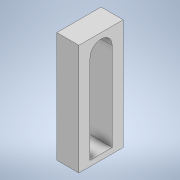
# Autodesk Inventor part: 뚫린 직육면체
Saved by Autodesk Inventor 2022 (Build 260153000, 153)
## iProperties
Created: 2022-10-28
Part Number: 뚫린 직육면체
Material: 일반
Document SubType Name: Modeling
Designer: gogin
Density: 1 g/cm^3
Appearance: 기본값
Author: gogin
Autodesk Inventor part; units mm, degrees
ref_plane "YZ Plane" through (0, 0, 0) normal (1, 0, 0) x (0, 1, 0)
ref_plane "XZ Plane" through (0, 0, 0) normal (0, 1, 0) x (-1, 0, 0)
ref_plane "XY Plane" through (0, 0, 0) normal (0, 0, 1) x (1, 0, 0)
sketch "스케치1" plane through (0, 0, 0) normal (1, 0, 0) x (0, 1, 0)
  line L0 (4.5, 0) -> (-0.5, 0)
  line L1 (-0.5, 0) -> (-0.5, -2)
  line L2 (-0.5, -2) -> (4.5, -2)
  line L3 (4.5, -2) -> (4.5, 0)
  point P0 (0, 0)
  dimension "d0" = 5
  dimension "d1" = 2
  dimension "d2" = 4.5
  dimension "d3" = 2
  constraints: 8 end point, 2 parallel, 1 horizontal, 1 perpendicular
  measures "d0" distance of L0.start L0.end
  measures "d1" distance of L2.end L0.start
  measures "d2" distance from line of point (0, 0) L3
  measures "d3" distance from line of L2 point (0, 0)
extrude "돌출1" add sketch "스케치1" along normal blind 1
sketch "스케치3" plane through (1, 0, 0) normal (1, 0, 0) x (0, 0, -1)
  line L0 (1, 4.25) -> (1, 4.25)
  line L1 (1.5, 3.75) -> (1.5, -0.25)
  line L2 (1.5, -0.25) -> (0.5, -0.25)
  line L3 (0.5, -0.25) -> (0.5, 3.75)
  arc A0 (1, 4.25) -> (0.5, 3.75) centre (1, 3.75) ccw
  arc A1 (1.5, 3.75) -> (1, 4.25) centre (1, 3.75) ccw
  point P0 (0, 0)
  point P1 (0.5, 4.25)
  point P2 (1.5, 4.25)
  dimension "d13" = 1
  dimension "d14" = 4.5
  dimension "d15" = 4.25
  dimension "d16" = 1.5
  dimension "d19" = 0.5
  constraints: 8 end point, 4 point on circle, 4 point on line, 4 tangent, 2 centre point, 2 parallel, 1 concentric, 1 horizontal, 1 perpendicular
  measures "d13" distance of point (0.5, 4.25) point (1.5, 4.25)
  measures "d14" distance of point (1.5, 4.25) L1.end
  measures "d15" distance from line of point (0, 0) L0
  measures "d16" distance from line of L1 point (0, 0)
  measures "d19" radius of A0
extrude "돌출2" cut sketch "스케치3" against normal blind 1
